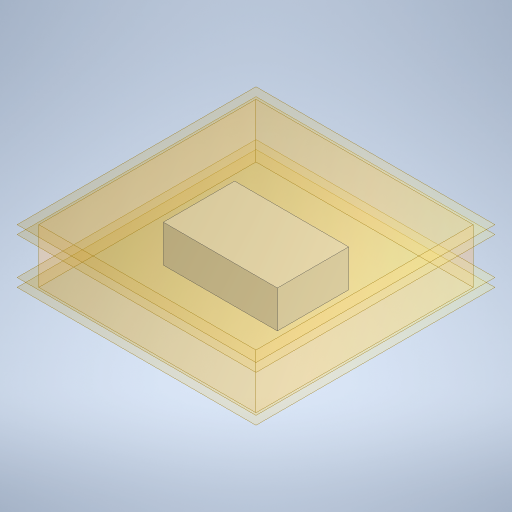
# Autodesk Inventor part: molde
Saved by Autodesk Inventor 2023.2 (Build 272271030, 271C)
## iProperties
Created: 2023-07-31
Part Number: molde
Material: Generic
Document SubType Name: Modeling
Designer: Cris Pat
Density: 1 g/cm^3
Appearance: Default
Author: Cris Pat
Autodesk Inventor part; units mm, degrees
ref_plane "YZ Plane" through (0, 0, 0) normal (1, 0, 0) x (0, 1, 0)
ref_plane "XZ Plane" through (0, 0, 0) normal (0, 1, 0) x (-1, 0, 0)
sketch "Sketch1" plane through (0, 0, 0) normal (0, 0, 1) x (1, 0, 0)
  line L0 (0, 76.2) -> (76.2, 76.2)
  line L1 (76.2, 76.2) -> (76.2, 0)
  line L2 (76.2, 0) -> (0, 0)
  line L3 (0, 0) -> (0, 76.2)
  dimension "d0" = 76.2
  dimension "d1" = 76.2
  constraints: 8 end point, 2 parallel, 1 coincident, 1 horizontal, 1 perpendicular
  measures "d0" distance of L1.end L2.end
  measures "d1" distance of L0.end L1.end
surface extrude "ExtrusionSrf1" sketch "Sketch1" against normal blind 19.05 shown yes curves L3 L0 L1 L2
ref_plane "Work Plane1" through (0, 0, -19.05) normal (0, 0, 1) x (1, 0, 0)
ref_plane "Work Plane2" through (0, 0, -3) normal (0, 0, 1) x (1, 0, 0)
ref_plane "Work Plane3" through (0, 0, -16.05) normal (0, 0, 1) x (1, 0, 0)
sketch "Sketch2" plane through (0, 0, -16.05) normal (0, 0, 1) x (1, 0, 0)
  line L0 (18.1, 25.6) -> (58.1, 25.6)
  line L1 (58.1, 25.6) -> (58.1, 50.6)
  line L2 (58.1, 50.6) -> (18.1, 50.6)
  line L3 (18.1, 50.6) -> (18.1, 25.6)
  line L4 (18.1, 25.6) -> (58.1, 50.6) construction
  line L5 (58.1, 25.6) -> (18.1, 50.6) construction
  point P0 (0, 0)
  point P1 (38.1, 38.1)
  dimension "d7" = 40
  dimension "d8" = 25
  dimension "d9" = 38.1
  dimension "d10" = 38.1
  constraints: 12 end point, 2 midpoint, 2 parallel, 1 horizontal, 1 perpendicular
  measures "d7" distance of L2.end L1.end
  measures "d8" distance of L1.end L0.end
  measures "d9" horizontal distance of point (0, 0) point (38.1, 38.1)
  measures "d10" horizontal distance of point (38.1, 38.1) point (0, 0)
extrude "Extrusion1" add sketch "Sketch2" along normal up to surface (13.05 mm away)
body "Solid1"
body "Srf1"
